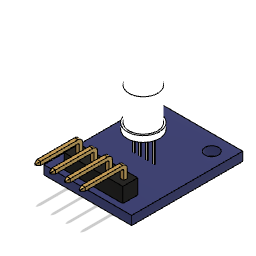
Led RGB for arduino (Autodesk Fusion 360 design; units mm, degrees)
Autodesk Fusion 360 part; units mm, degrees
note: some values were not read from the file. Chosen so that the rebuilt part matches the saved one: which bodies a step acts on.
sketch "Sketch1" plane through (0, 0, 0) normal (0, 1, 0) x (1, 0, 0)
  line L0 (-7.5, 9.5) -> (7.5, 9.5)
  line L1 (7.5, 9.5) -> (7.5, -9.5)
  line L2 (7.5, -9.5) -> (-7.5, -9.5)
  line L3 (-7.5, -9.5) -> (-7.5, 9.5)
  dimension "d1" = 15
  dimension "d2" = 19
  dimension "d3" = 7.5
  dimension "d4" = 9.5
  constraint horizontal L0
  constraint vertical L1
  constraint horizontal L2
  constraint vertical L3
  measures "d1" horizontal distance of L0.start L0.end
  measures "d2" vertical distance of L0.end L1.end
  measures "d3" horizontal distance of origin L0.start
  measures "d4" vertical distance of origin L0.start
extrude "Extrude1" add sketch "Sketch1" along normal blind 1.5 makes body 1
ref_plane "WorkPlane1" through (0, 0.75, 0) normal (0, 0, 1) x (1, 0, 0)
sketch "Sketch2" plane through (0, 0.75, 0) normal (0, 0, 1) x (1, 0, 0)
  line L0 (0, 5) -> (-2.75, 5)
  line L1 (-2.75, 5) -> (-2.75, 6)
  line L2 (-2.45, 11.55) -> (-2.45, 6)
  arc A0 (0, 14) -> (-2.45, 11.55) centre (0, 11.55) ccw
  line L3 (-2.75, 6) -> (-2.45, 6)
  line L4 (0, 14) -> (0, 5)
  dimension "d7" = 4.9
  dimension "d10" = 5
  dimension "d11" = 2.75
  dimension "d12" = 6.55
  dimension "d13" = 2.75
  constraint horizontal L3
  constraint horizontal L0
  constraint vertical L1
  constraint vertical L2
  constraint tangent L2 A0
  measures "d7" diameter of A0
  measures "d10" vertical distance of origin L0.end
  measures "d11" horizontal distance of origin L0.end
  measures "d12" vertical distance of A0.centre L0.end
  measures "d13" horizontal distance of A0.centre L1.end
revolve "Revolve1" add sketch "Sketch2" angle 360 about axis through (0, 1.75, 0) along (0, 1, 0) separate body makes body 2
sketch "Sketch3" plane through (0, 0.75, 0) normal (0, 0, 1) x (1, 0, 0)
sketch "Sketch4" plane through (0, 5.75, 0) normal (0, -1, 0) x (1, 0, 0)
  circle A0 centre (0, 0) radius 2.75
  line L0 (-1.8297, 0) -> (-1.5038, 0)
  line L1 (-1.5038, 0) -> (-1.5038, -0.1423)
  line L2 (-1.5038, -0.1423) -> (-1.8297, -0.1423)
  line L3 (-1.8297, -0.1423) -> (-1.8297, 0)
  line L4 (-0.8297, 0) -> (-0.5038, 0)
  line L5 (-0.8297, -0.1423) -> (-0.8297, 0)
  line L6 (-0.5038, 0) -> (-0.5038, -0.1423)
  line L7 (-0.5038, -0.1423) -> (-0.8297, -0.1423)
  line L8 (0.6962, 0) -> (0.6962, -0.1423)
  line L9 (0.3703, 0) -> (0.6962, 0)
  line L10 (0.6962, -0.1423) -> (0.3703, -0.1423)
  line L11 (0.3703, -0.1423) -> (0.3703, 0)
  line L12 (1.8962, 0) -> (1.8962, -0.1423)
  line L13 (1.8962, -0.1423) -> (1.5703, -0.1423)
  line L14 (1.5703, -0.1423) -> (1.5703, 0)
  line L15 (1.5703, 0) -> (1.8962, 0)
  constraint horizontal L0
  constraint vertical L1
  constraint horizontal L2
  constraint vertical L3
  constraint horizontal L4
  constraint vertical L6
  constraint horizontal L7
  constraint vertical L5
  constraint horizontal L9
  constraint vertical L8
  constraint horizontal L10
  constraint vertical L11
  constraint horizontal L15
  constraint vertical L12
  constraint horizontal L13
  constraint vertical L14
extrude "Extrude2" add sketch "Sketch4" along normal blind 6 contours L0 L1 L2 L3 | L4 L5 L6 L7 | L8 L9 L10 L11 | L12 L13 L14 L15 bodies 2
sketch "Sketch5" plane through (0, 1.5, 0) normal (0, 1, 0) x (-1, 0, 0)
  line L0 (7.5, 9.5) -> (-7.5, 9.5)
  line L1 (-7.5, 9.5) -> (-7.5, -9.5)
  line L2 (-7.5, -9.5) -> (7.5, -9.5)
  line L3 (7.5, -9.5) -> (7.5, 9.5)
  line L4 (5, 5.96) -> (-5, 5.96)
  line L5 (-5, 5.96) -> (-5, 8.5)
  line L6 (-5, 8.5) -> (5, 8.5)
  line L7 (5, 8.5) -> (5, 5.96)
  dimension "d17" = 2.54
  dimension "d18" = 10
  dimension "d19" = 5
  dimension "d20" = 1
  constraint horizontal L4
  constraint vertical L5
  constraint horizontal L6
  constraint vertical L7
  measures "d17" vertical distance of L4.end L5.end
  measures "d18" horizontal distance of L4.start L4.end
  measures "d19" horizontal distance of origin L4.start
  measures "d20" vertical distance of L0.start L6.end
extrude "Extrude3" add sketch "Sketch5" along normal blind 2.54 contours L4 L5 L6 L7 bodies 1
sketch "Sketch6" plane through (0, 4.04, 0) normal (0, 1, 0) x (-1, 0, 0)
  line L0 (5, 8.5) -> (-5, 8.5)
  line L1 (-5, 8.5) -> (-5, 5.96)
  line L2 (-5, 5.96) -> (5, 5.96)
  line L3 (5, 5.96) -> (5, 8.5)
  line L4 (4.03, 6.93) -> (3.43, 6.93)
  line L5 (3.43, 6.93) -> (3.43, 7.53)
  line L6 (3.43, 7.53) -> (4.03, 7.53)
  line L7 (4.03, 7.53) -> (4.03, 6.93)
  line L8 (1.49, 6.93) -> (0.89, 6.93)
  line L9 (1.49, 7.53) -> (1.49, 6.93)
  line L10 (0.89, 7.53) -> (1.49, 7.53)
  line L11 (0.89, 6.93) -> (0.89, 7.53)
  line L12 (-1.05, 6.93) -> (-1.65, 6.93)
  line L13 (-1.05, 7.53) -> (-1.05, 6.93)
  line L14 (-1.65, 7.53) -> (-1.05, 7.53)
  line L15 (-1.65, 6.93) -> (-1.65, 7.53)
  line L16 (-3.59, 6.93) -> (-4.19, 6.93)
  line L17 (-3.59, 7.53) -> (-3.59, 6.93)
  line L18 (-4.19, 7.53) -> (-3.59, 7.53)
  line L19 (-4.19, 6.93) -> (-4.19, 7.53)
  dimension "d23" = 0.6
  dimension "d24" = 0.6
  dimension "d25" = 0.97
  dimension "d26" = 0.97
  dimension "d29" = -2.54
  dimension "d30" = 0
  constraint horizontal L4
  constraint vertical L5
  constraint horizontal L6
  constraint vertical L7
  measures "d23" distance of L4.start L4.end
  measures "d24" distance of L4.start L6.end
  measures "d25" vertical distance of L2.end L4.start
  measures "d26" horizontal distance of L2.end L4.start
ref_plane "WorkPlane2" through (-3.73, 2.77, 7.23) normal (-1, 0, 0) x (0, 0, 1)
sketch "Sketch8" plane through (-3.73, 2.77, 7.23) normal (-1, 0, 0) x (0, 0, -1)
  line L0 (0.3, -1.27) -> (-0.3, -1.27)
  line L1 (0, -1.27) -> (0, -2.77)
  line L2 (-0.5, -3.27) -> (-7.5, -3.27)
  arc A0 (-0.5, -3.27) -> (0, -2.77) centre (-0.5, -2.77) ccw
  point P0 (0, -3.27)
  dimension "d32" = 7.5
  dimension "d33" = 0.5
  constraint midpoint L0 L1.start
  constraint coincident P0 L1
  constraint coincident P0 L2
  constraint tangent L1 A0
  constraint tangent L2 A0
  measures "d32" distance of P0 L2.end
  measures "d33" radius of A0
sweep "Sweep1" add profiles "Sketch6" path "Sketch8" along L1 A0 L2 section 1 contours L4 L5 L6 L7 separate body makes body 3
chamfer "Chamfer1" distance 0.2 distance2 0.6 4 edges at (-3.73, 6.34, 14.73) (-4.03, 6.04, 14.73) (-3.73, 5.74, 14.73) (-3.43, 6.04, 14.73) measured on face at (-3.63, 5.94, 14.73) measured on face at (-3.63, 5.94, 14.73) measured on face at (-3.63, 5.94, 14.73) measured on face at (-3.63, 5.94, 14.73) on bodies 3
pattern_linear "R-Pattern1" count 4 spacing 2.54 along (1, 0, 0) of bodies 3 makes body 4 at (-0.89, 5.94, 11.9967) makes body 5 at (1.65, 5.94, 11.9967) makes body 6 at (4.19, 5.94, 11.9967)
split "Split1" by plane through (0, 5.75, 0) normal (0, -1, 0) bodies 2 makes body 7 at (-1.6124, 3.75, -0.1423) makes body 8 at (-0.6124, 3.75, -0.1423) makes body 9 at (0.4789, 3.75, 0) makes body 10 at (1.6789, 3.75, 0)
split "Split2" by plane through (0, 1.5, 0) normal (0, 1, 0) bodies 1 makes body 11 at (1.6667, 2.3467, 8.5)
sketch "Sketch9" plane through (0, 1.5, 0) normal (0, 1, 0) x (-1, 0, 0)
  line L0 (7.5, 9.5) -> (-7.5, 9.5)
  line L1 (-7.5, 9.5) -> (-7.5, -9.5)
  line L2 (-7.5, -9.5) -> (7.5, -9.5)
  line L3 (7.5, -9.5) -> (7.5, 9.5)
  line L4 (0, -11.7248) -> (0, 3) construction
  circle A0 centre (4.85, -6.85) radius 1.15
  circle A1 centre (-4.85, -6.85) radius 1.15
  dimension "d46" = 2.3
  dimension "d47" = 1.5
  dimension "d48" = 1.5
  constraint perpendicular L2 L4
  constraint coincident origin L4
  constraint symmetric L4 A0 A1
  measures "d46" diameter of A0
  measures "d47" distance of L2 A0
  measures "d48" distance of L3 A0
extrude "Extrude4" cut sketch "Sketch9" against normal blind 3 contours A0 | A1 bodies 1
equation "d3 = d1 / 2"
equation "d4 = d2 / 2"
equation "d8 = 5.5 mm"
equation "d11 = d8 / 2"
equation "d12 = 9 mm - ( d7 / 2 )"
equation "d13 = d11"
equation "d19 = d18 / 2"
equation "d25 = ( ( 2.54 / 2 ) * 1 mm ) - ( d24 / 2 )"
equation "d26 = d25"
equation "d31 = ( -2.54 / 2 ) * 1 mm"
